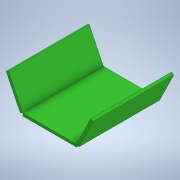
# Autodesk Inventor part: buttons2_PCBs
Saved by Autodesk Inventor 2020 (Build 240168000, 168)
## iProperties
Created: 2019-11-18
Part Number: buttons2_PCBs
Material: Generic
Document SubType Name: Modeling
Designer: suchanek
Density: 1 g/cm^3
Appearance: Default
Author: suchanek
Autodesk Inventor part; units mm, degrees
ref_plane "YZ Plane" through (0, 0, 0) normal (1, 0, 0) x (0, 1, 0)
ref_plane "XZ Plane" through (0, 0, 0) normal (0, 1, 0) x (-1, 0, 0)
ref_plane "XY Plane" through (0, 0, 0) normal (0, 0, 1) x (1, 0, 0)
sketch "Sketch1" plane through (0, 0, 0) normal (0, 0, 1) x (1, 0, 0)
  line L0 (0, 0) -> (-20, 0)
  line L1 (-20, 0) -> (-20, -1)
  line L2 (-20, -1) -> (0, -1)
  line L3 (0, -1) -> (0, 0)
  line L4 (0, 0) -> (5.2584, 10.7865)
  line L5 (5.2584, 10.7865) -> (6.1573, 10.3483)
  line L6 (6.1573, 10.3483) -> (0.8989, -0.4382)
  line L7 (0.8989, -0.4382) -> (0, 0)
  line L8 (-20, 0) -> (-25.2584, 10.7865)
  line L9 (-25.2584, 10.7865) -> (-26.1573, 10.3483)
  line L10 (-26.1573, 10.3483) -> (-20.8989, -0.4382)
  line L11 (-20.8989, -0.4382) -> (-20, 0)
  circle A0 centre (-10, 16) radius 16
  dimension "d0" = 20
  dimension "d1" = 1
  dimension "d2" = 1
  dimension "d3" = 1
  dimension "d4" = 32
  dimension "d5" = 12
  dimension "d6" = 12
  constraints: 24 end point, 6 parallel, 3 perpendicular, 3 tangent, 1 centre point, 1 horizontal, 1 horizontal alignment
  measures "d0" distance of L2.end L1.end
  measures "d1" distance of L1.end L0.end
  measures "d2" distance of L8.end L9.end
  measures "d3" distance of L4.end L5.end
  measures "d4" diameter of A0
  measures "d5" distance of L5.end L6.end
  measures "d6" distance of L9.end L10.end
extrude "Extrusion1" add sketch "Sketch1" along normal blind 30 contours L3 L2 L1 L0 | L4 L5 L6 L7 | L11 L10 L9 L8
body "Solid1"
